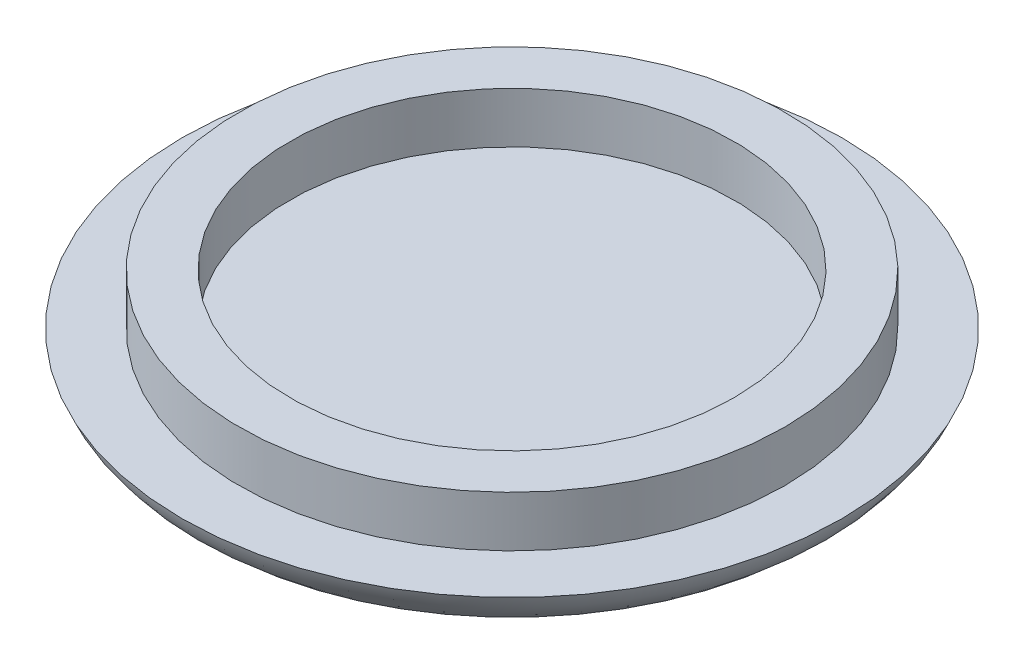
hubcap_rear (Autodesk Fusion 360 design; units mm, degrees)
part number: 2026-03-29-10-00-40-740
Autodesk Fusion 360 part; units mm, degrees
sketch "Sketch1" plane through (0, 0, 0) normal (0, 0, 1) x (1, 0, 0)
  circle A0 centre (0, 0) radius 13
  dimension "d89" = 26
  constraint coincident A0.centre origin
  measures "d89" diameter of A0
extrude "Extrude1" add sketch "Sketch1" along normal blind 2
fillet "Fillet1" radius 3 1 edges at (-12.1203, -4.701, 2)
sketch "Sketch3" plane through (0, 0, 0) normal (0, 0, 1) x (1, 0, 0)
  circle A0 centre (0, 0) radius 3.75
  dimension "d1" = 7.5
  constraint coincident A0.centre origin
  measures "d1" diameter of A0
move_body "Move1" bodies 1 to x (1, 0, 0) y (0, 1, 0) z (0, 0, 1) at (0, 3, 0)
move_body "Move2" bodies 1 to x (1, 0, 0) y (0, 1, 0) z (0, 0, 1) at (0, 0, -3)
move_body "Move3" bodies 1 to x (-1, 0, 0) y (0, 1, 0) z (0, 0, -1) at (0, -3, -1)
sketch "Sketch4" plane through (0, 0, 2) normal (0, 0, 1) x (-1, 0, 0)
  circle A0 centre (0, 0) radius 13
  circle A1 centre (0, 0) radius 8.75
  circle A2 centre (0, 0) radius 10.75
  dimension "d4" = 17.5
  dimension "d5" = 21.5
  constraint coincident A0.centre A1.centre
  constraint concentric A0 A2
  measures "d4" diameter of A1
  measures "d5" diameter of A2
extrude "Extrude4" add sketch "Sketch4" along normal blind 2 contours A2
